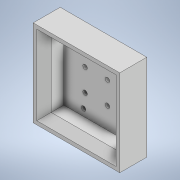
# Autodesk Inventor part: one-square
Saved by Autodesk Inventor 2021 (Build 250183000, 183)
## iProperties
Created: 2020-12-08
Part Number: one-square
Material: Generic
Document SubType Name: Modeling
Designer: Luke Kamols
Density: 1 g/cm^3
Appearance: Default
Author: Luke Kamols
Autodesk Inventor part; units mm, degrees
ref_plane "YZ Plane" through (0, 0, 0) normal (1, 0, 0) x (0, 1, 0)
ref_plane "XZ Plane" through (0, 0, 0) normal (0, 1, 0) x (-1, 0, 0)
ref_plane "XY Plane" through (0, 0, 0) normal (0, 0, 1) x (1, 0, 0)
sketch "Sketch1" plane through (0, 0, 0) normal (0, 0, 1) x (1, 0, 0)
  line L0 (0, 0) -> (48, 0)
  line L1 (48, 0) -> (48, 48)
  line L2 (48, 48) -> (0, 48)
  line L3 (0, 48) -> (0, 0)
  dimension "d0" = 48
  dimension "d1" = 48
  constraints: 8 end point, 2 parallel, 1 horizontal, 1 perpendicular
  measures "d0" distance of L2.end L1.end
  measures "d1" distance of L1.end L0.end
extrude "Extrusion1" add sketch "Sketch1" along normal blind 15
sketch "Sketch2" plane through (0, 0, 15) normal (0, 0, 1) x (1, 0, 0)
  line L0 (6, 6) -> (42, 6)
  line L1 (42, 6) -> (42, 42)
  line L2 (42, 42) -> (6, 42)
  line L3 (6, 42) -> (6, 6)
  point P0 (0, 0)
  dimension "d6" = 36
  dimension "d7" = 36
  constraints: 8 end point, 2 parallel, 1 horizontal, 1 perpendicular
  measures "d6" distance of L2.end L1.end
  measures "d7" distance of L1.end L0.end
extrude "Extrusion2" cut sketch "Sketch2" against normal blind 11
chamfer "Chamfer1" distance 4 angle 45 4 edges at (42, 24, 15) (24, 42, 15) (6, 24, 15) (24, 6, 15)
sketch "Sketch3" plane through (0, 0, 4) normal (0, 0, 1) x (1, 0, 0)
  line L0 (0, 0) -> (24, 0)
  line L1 (0, 24) -> (0, 0)
  line L2 (46, 46) -> (2, 46) projected
  line L3 (26.6, 24) -> (26.6, 24.8)
  line L4 (26.6, 24.8) -> (30.2, 24.8)
  line L5 (30.2, 24.8) -> (30.2, 23.2)
  line L6 (30.2, 23.2) -> (26.6, 23.2)
  line L7 (24, 21.4) -> (24.8, 21.4)
  line L8 (24.8, 21.4) -> (24.8, 17.8)
  line L9 (24.8, 17.8) -> (23.2, 17.8)
  line L10 (23.2, 17.8) -> (23.2, 21.4)
  line L11 (21.4, 23.2) -> (17.8, 23.2)
  line L12 (17.8, 23.2) -> (17.8, 24.8)
  line L13 (17.8, 24.8) -> (21.4, 24.8)
  line L14 (24, 26.6) -> (24.8, 26.6)
  line L15 (24.8, 26.6) -> (24.8, 30.2)
  line L16 (24.8, 30.2) -> (23.2, 30.2)
  line L17 (23.2, 30.2) -> (23.2, 26.6)
  line L18 (48, 48) -> (0, 48) projected
  line L19 (0, 48) -> (0, 0) projected
  circle A0 centre (38.1421, 31.0711) radius 1.25
  circle A1 centre (16.9289, 9.8579) radius 1.25
  line L20 (21.4, 23.2) -> (21.4, 24.8)
  line L21 (23.2, 26.6) -> (24, 26.6)
  line L22 (26.6, 23.2) -> (26.6, 24)
  line L23 (23.2, 21.4) -> (24, 21.4)
  circle A2 centre (26.6, 21.4) radius 1.25
  circle A3 centre (21.4, 26.6) radius 1.25
  circle A4 centre (26.6, 26.6) radius 1.25
  circle A5 centre (21.4, 21.4) radius 1.25
  line L24 (24, 24) -> (30.2, 24)
  circle A6 centre (30.2, 30.2) radius 1.25
  circle A7 centre (17.8, 30.2) radius 1.25
  circle A8 centre (17.8, 17.8) radius 1.25
  circle A9 centre (30.2, 17.8) radius 1.25
  circle A10 centre (9.8579, 9.8579) radius 1.25
  circle A11 centre (38.1421, 38.1421) radius 1.25
  point P0 (48, 0)
  dimension "d21" = 0.8
  dimension "d22" = 3.6
  dimension "d23" = 1.6
  dimension "d25" = 3.6
  dimension "d26" = 1.6
  dimension "d27" = 3.6
  dimension "d28" = 1.6
  dimension "d30" = 1.6
  dimension "d62" = 2.5
  dimension "d63" = 2.5
  dimension "d64" = 2.5
  dimension "d65" = 2.5
  dimension "d66" = 2.5
  dimension "d67" = 2.5
  constraints: 44 end point, 12 centre point, 8 point on line, 5 perpendicular, 1 horizontal, 1 midpoint, 1 vertical
  measures "d21" distance of L3.start L3.end
  measures "d22" distance of L3.end L4.end
  measures "d23" distance of L4.end L5.end
  measures "d25" distance of L7.end L8.end
  measures "d26" distance of L8.end L9.end
  measures "d27" distance of L11.start L11.end
  measures "d28" distance of L11.end L12.end
  measures "d30" distance of L15.end L16.end
  measures "d62" diameter of A6
  measures "d63" diameter of A7
  measures "d64" diameter of A8
  measures "d65" diameter of A9
  measures "d66" diameter of A10
  measures "d67" diameter of A11
extrude "Extrusion4" cut sketch "Sketch3" against normal blind 5 contours A0 | A1 | A6 | A7 | A8 | A9
body "Solid1"
